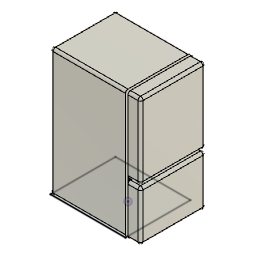
rgiro_generic_refrigerator (Autodesk Fusion 360 design; units mm, degrees)
Autodesk Fusion 360 part; units mm, degrees
sketch "Sketch1" plane through (0, 0, 0) normal (0, 0, 1) x (1, 0, 0)
  line L0 (240, 260) -> (-360, 260)
  line L1 (-360, 260) -> (-360, -260)
  line L2 (-360, -260) -> (240, -260)
  line L3 (240, -260) -> (240, 260)
  dimension "d7" = 520
  dimension "d8" = 600
  dimension "d10" = 260
  dimension "d11" = 360
  constraint horizontal L0
  constraint vertical L1
  constraint horizontal L2
  constraint vertical L3
  measures "d7" distance of L0.start L2.end
  measures "d8" distance of L0.start L0.end
  measures "d10" distance of origin L0
  measures "d11" distance of origin L1
extrude "Extrude2" add sketch "Sketch1" along normal blind 1020 makes body 1
sketch "Sketch3" plane through (240, 0, 0) normal (1, 0, 0) x (0, 1, 0)
  line L0 (-260, 0) -> (260, 0)
  line L1 (260, 0) -> (260, 1020)
  line L2 (260, 1020) -> (-260, 1020)
  line L3 (-260, 1020) -> (-260, 0)
  line L4 (-240, 20) -> (240, 20)
  line L5 (240, 20) -> (240, 1000)
  line L6 (240, 1000) -> (-240, 1000)
  line L7 (-240, 1000) -> (-240, 20)
  dimension "d14" = -20
extrude "Extrude3" add sketch "Sketch3" along normal blind 20 separate body contours L4 L5 L6 L7 makes body 2
sketch "Sketch4" plane through (260, 0, 0) normal (1, 0, 0) x (0, 1, 0)
  line L0 (-240, 1000) -> (-240, 20)
  line L1 (-240, 20) -> (240, 20)
  line L2 (240, 20) -> (240, 1000)
  line L3 (240, 1000) -> (-240, 1000)
  line L4 (-260, 0) -> (260, 0)
  line L5 (260, 0) -> (260, 1020)
  line L6 (260, 1020) -> (-260, 1020)
  line L7 (-260, 1020) -> (-260, 0)
  line L8 (-260, 0) -> (260, 0)
  line L9 (260, 0) -> (260, 400)
  line L10 (260, 400) -> (-260, 400)
  line L11 (-260, 400) -> (-260, 0)
  line L12 (-260, 1020) -> (260, 1020)
  line L13 (260, 1020) -> (260, 420)
  line L14 (260, 420) -> (-260, 420)
  line L15 (-260, 420) -> (-260, 1020)
  dimension "d17" = 400
  dimension "d18" = 600
  constraint horizontal L8
  constraint vertical L9
  constraint horizontal L10
  constraint vertical L11
  constraint coincident L5 L9.end
  constraint coincident L4.start L7.end
  constraint horizontal L12
  constraint vertical L13
  constraint horizontal L14
  constraint vertical L15
  constraint coincident L6.end L7.start
  constraint collinear L5 L13
  measures "d17" distance of L8 L10
  measures "d18" distance of L5.end L13.end
extrude "Extrude4" add sketch "Sketch4" along normal blind 100 separate body contours L0 L2 L3 L14 | L0 L2 L3 L5 L6 L7 L12 L13 L14 L15 | L0 L1 L2 L10 | L0 L1 L2 L4 L5 L7 L8 L9 L10 L11 makes body 3 at (260, -86.6667, 266.6667) makes body 4 at (260, -86.6667, 820)
fillet "Fillet1" radius 20 12 edges at (-60, -260, 0) (-60, 260, 0) (-60, 260, 1020) (-60, -260, 1020) (310, -260, 400) (310, -260, 0) (310, 260, 0) (310, 260, 400) (310, -260, 1020) (310, 260, 1020) (310, 260, 420) (310, -260, 420) 3 faces at (-360, 86.6667, 340) (360, -86.6667, 266.6667) (360, 86.6667, 620) on bodies 1 3 4
fillet "Fillet2" radius 20 4 edges at (250, 240, 1000) (250, -240, 1000) (250, -240, 20) (250, 240, 20) on bodies 2
